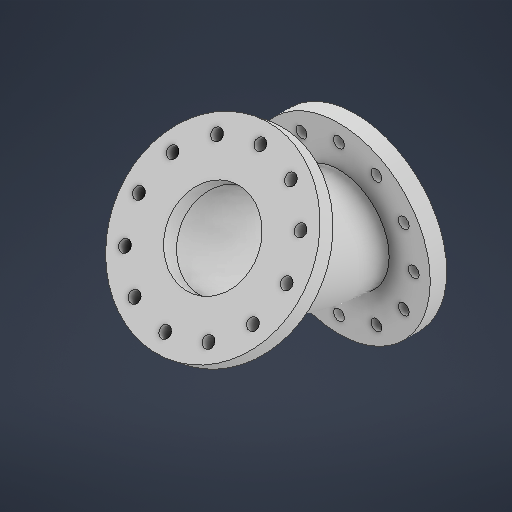
# Autodesk Inventor part: crazy
Saved by Autodesk Inventor 2026.2 (Build 302298010, 298A)
## iProperties
Created: 2026-03-28
Part Number: crazy
Material: Generic
Document SubType Name: Modeling
Designer: munis
Density: 1 g/cm^3
Appearance: Default
Author: munis
Autodesk Inventor part; units mm, degrees
ref_plane "YZ Plane" through (0, 0, 0) normal (1, 0, 0) x (0, 1, 0)
ref_plane "XY Plane" through (0, 0, 0) normal (0, 0, 1) x (1, 0, 0)
sketch "Sketch2" plane through (0, 0, 0) normal (0, 0, 1) x (1, 0, 0)
  circle A0 centre (0, 0) radius 61
  circle A1 centre (0, 0) radius 28
  line L0 (0, 68.8089) -> (0, -61.0943)
  line L1 (-74.2561, 0) -> (92.1735, 0)
  circle A2 centre (0, 50) radius 3.665
  circle A3 centre (-25, 43.3013) radius 3.665
  circle A4 centre (-43.3013, 25) radius 3.665
  circle A5 centre (-50, 0) radius 3.665
  circle A6 centre (-43.3013, -25) radius 3.665
  circle A7 centre (-25, -43.3013) radius 3.665
  circle A8 centre (0, -50) radius 3.665
  circle A9 centre (25, -43.3013) radius 3.665
  circle A10 centre (43.3013, -25) radius 3.665
  circle A11 centre (50, 0) radius 3.665
  circle A12 centre (43.3013, 25) radius 3.665
  circle A13 centre (25, 43.3013) radius 3.665
  dimension "d0" = 122
  dimension "d1" = 56
  dimension "d2" = 7.33
  dimension "d4" = 50
  dimension "d7" = 360
  constraints: 14 centre point, 4 end point, 2 coincident, 1 horizontal, 1 point on line, 1 vertical, 25 other
  measures "d0" diameter of A0
  measures "d1" diameter of A1
  measures "d2" diameter of A2
  measures "d4" distance of A0.centre A2.centre
extrude "Extrusion1" add sketch "Sketch2" along normal blind 11 contours L1 A11 A1 L0 A2 A0 | A0 L0 A8 A1 L1 A11 | L0 A2 A1 L1 A5 A0 | A0 L1 A5 A1 L0 A8
ref_plane "Work Plane1" through (0, 145, 0) normal (0, 1, 0) x (-1, 0, 0)
sketch "Sketch4" plane through (0, 0, 0) normal (0, 0, -1) x (-1, 0, 0)
  circle A0 centre (0, 0) radius 28
  circle A1 centre (0, 0) radius 33.5
  line L0 (-79.8111, 140.7115) -> (80.5184, 140.7115) construction
  dimension "d12" = 56
  dimension "d13" = 67
  constraints: 2 centre point, 2 coincident, 2 end point, 1 horizontal
  measures "d12" diameter of A0
  measures "d13" diameter of A1
revolve "Revolution1" add sketch "Sketch4" angle 38 about axis through (79.8111, 140.7115, 0) along (-1, 0, 0)
sketch "Sketch5" plane through (0, 29.8293, 86.6306) normal (0, 0.6157, 0.788) x (1, 0, 0)
  circle A0 centre (0, 0) radius 61
  circle A1 centre (0, 0) radius 28
  line L0 (25.8703, 42.9334) -> (25.8703, -86.9698)
  line L1 (-48.3858, -25.8755) -> (118.0439, -25.8755)
  circle A2 centre (25.8703, 42.787) radius 3.665
  circle A3 centre (1.0109, 49.9898) radius 3.665
  circle A4 centre (-24.1194, 43.7979) radius 3.665
  circle A5 centre (-42.787, 25.8703) radius 3.665
  circle A6 centre (-49.9898, 1.0109) radius 3.665
  circle A7 centre (-43.7979, -24.1194) radius 3.665
  circle A8 centre (-25.8703, -42.787) radius 3.665
  circle A9 centre (-1.0109, -49.9898) radius 3.665
  circle A10 centre (24.1194, -43.7979) radius 3.665
  circle A11 centre (42.787, -25.8703) radius 3.665
  circle A12 centre (49.9898, -1.0109) radius 3.665
  circle A13 centre (43.7979, 24.1194) radius 3.665
  point P0 (0, 29.8293)
  dimension "d17" = 122
  dimension "d18" = 56
  dimension "d19" = 7.33
  dimension "d20" = 50
  dimension "d21" = 360
  constraints: 14 centre point, 4 end point, 2 coincident, 1 horizontal, 1 point on line, 1 vertical, 25 other
  measures "d17" diameter of A0
  measures "d18" diameter of A1
  measures "d19" diameter of A2
  measures "d20" distance of A0.centre A2.centre
extrude "Extrusion2" add sketch "Sketch5" along normal blind 11 contours L1 A1 L0 | A0 L1 A11 L0 A10 | L0 A10 L1 A11 A0 picked at (22.9817, -20.4121)
body "Solid1"
